init v9 (Autodesk Fusion 360 design; units mm, degrees)
Autodesk Fusion 360 part; units mm, degrees
sketch "Sketch1" plane through (0, 0, 0) normal (0, 0, 1) x (1, 0, 0)
  circle A0 centre (0, 0) radius 15
  circle A1 centre (0, 0) radius 20
  constraint coincident A0.centre A1.centre
extrude "Extrude1" add sketch "Sketch1" against normal blind 80 makes body 1
sketch "Sketch2" plane through (0, 0, 0) normal (0, 0, 1) x (1, 0, 0)
  circle A0 centre (0, 0) radius 15
  circle A1 centre (0, 0) radius 20
  circle A2 centre (0, 0) radius 50
  dimension "d5" = 100
  constraint concentric A0 A2
  measures "d5" diameter of A2
extrude "Extrude2" add sketch "Sketch2" along normal blind 10 separate body contours A2 makes body 2
extrude "Extrude3" add 1 faces at (39.7394, -3.4777, 10) along direction (0, 0, 1) blind 10 on bodies 2 bodies 2
chamfer "Chamfer1" distance 20 angle 45 1 edges at (-18.6465, 7.2323, 20) on bodies 2
sketch "Sketch3" plane through (0, 0, 20) normal (0, 0, 1) x (1, 0, 0)
  circle A0 centre (0, 0) radius 50
  circle A1 centre (0, 0) radius 40
  circle A2 centre (0, 0) radius 50
  constraint concentric A0 A2
extrude "Extrude4" add sketch "Sketch3" along normal blind 15 separate body contours A0 A2 | A1 makes body 3
sketch "Sketch4" plane through (0, 0, 20) normal (0, 0, -1) x (-1, 0, 0)
  circle A0 centre (0, 0) radius 50
  circle A1 centre (0, 0) radius 32.5
  dimension "d13" = 65
  constraint concentric A0 A1
  measures "d13" diameter of A1
extrude "Extrude5" add sketch "Sketch4" along normal blind 20 separate body contours A1 makes body 4
chamfer "Chamfer2" distance 20 angle 45 1 edges at (30.3006, -11.7525, 0) on bodies 4
sketch "Sketch5" plane through (0, 0, 35) normal (0, 0, 1) x (1, 0, 0)
  circle A0 centre (0, 0) radius 50
  circle A1 centre (35, 0) radius 1.5
  circle A2 centre (32.3358, 13.3939) radius 1.5
  circle A3 centre (24.7487, 24.7487) radius 1.5
  circle A4 centre (13.3939, 32.3358) radius 1.5
  circle A5 centre (0, 35) radius 1.5
  circle A6 centre (-13.3939, 32.3358) radius 1.5
  circle A7 centre (-24.7487, 24.7487) radius 1.5
  circle A8 centre (-32.3358, 13.3939) radius 1.5
  circle A9 centre (-35, 0) radius 1.5
  circle A10 centre (-32.3358, -13.3939) radius 1.5
  circle A11 centre (-24.7487, -24.7487) radius 1.5
  circle A12 centre (-13.3939, -32.3358) radius 1.5
  circle A13 centre (0, -35) radius 1.5
  circle A14 centre (13.3939, -32.3358) radius 1.5
  circle A15 centre (24.7487, -24.7487) radius 1.5
  circle A16 centre (32.3358, -13.3939) radius 1.5
  dimension "d18" = 3
  measures "d18" diameter of A1
extrude "Extrude6" cut sketch "Sketch5" against normal blind 70 contours A1 | A2 | A3 | A4 | A5 | A6 | A7 | A8 | A9 | A10 | A11 | A12 | A13 | A14 | A15 | A16 bodies 3
sketch "Sketch6" plane through (0, 0, 0) normal (0, 0, -1) x (-1, 0, 0)
  circle A0 centre (0, 0) radius 20
  circle A1 centre (0, 0) radius 50
  circle A2 centre (0, 0) radius 22.5
  dimension "d23" = 45
  constraint concentric A0 A2
  measures "d23" diameter of A2
extrude "Extrude7" add sketch "Sketch6" along normal blind 10 separate body contours A2 makes body 5
sketch "Sketch7" plane through (0, 0, 35) normal (0, 0, 1) x (1, 0, 0)
  circle A0 centre (0, -35) radius 1.5
  circle A1 centre (35, 0) radius 1.5
  circle A2 centre (0, 35) radius 1.5
  circle A3 centre (-35, 0) radius 1.5
  circle A4 centre (-32.3358, 13.3939) radius 1.5
  circle A5 centre (13.3939, 32.3358) radius 1.5
  circle A6 centre (32.3358, -13.3939) radius 1.5
  circle A7 centre (-13.3939, -32.3358) radius 1.5
  circle A8 centre (13.3939, -32.3358) radius 1.5
  circle A9 centre (32.3358, 13.3939) radius 1.5
  circle A10 centre (-13.3939, 32.3358) radius 1.5
  circle A11 centre (-32.3358, -13.3939) radius 1.5
  circle A12 centre (-24.7487, 24.7487) radius 1.5
  circle A13 centre (24.7487, 24.7487) radius 1.5
  circle A14 centre (24.7487, -24.7487) radius 1.5
  circle A15 centre (-24.7487, -24.7487) radius 1.5
  circle A16 centre (0, 0) radius 50
  circle A17 centre (0, 43.25) radius 4
sketch "Sketch8" plane through (0, 0, 20) normal (0, 0, -1) x (-1, 0, 0)
  circle A0 centre (0, -35) radius 1.5
  circle A1 centre (-35, 0) radius 1.5
  circle A2 centre (0, 35) radius 1.5
  circle A3 centre (35, 0) radius 1.5
  circle A4 centre (32.3358, 13.3939) radius 1.5
  circle A5 centre (-13.3939, 32.3358) radius 1.5
  circle A6 centre (-32.3358, -13.3939) radius 1.5
  circle A7 centre (13.3939, -32.3358) radius 1.5
  circle A8 centre (-13.3939, -32.3358) radius 1.5
  circle A9 centre (-32.3358, 13.3939) radius 1.5
  circle A10 centre (13.3939, 32.3358) radius 1.5
  circle A11 centre (32.3358, -13.3939) radius 1.5
  circle A12 centre (24.7487, 24.7487) radius 1.5
  circle A13 centre (-24.7487, 24.7487) radius 1.5
  circle A14 centre (-24.7487, -24.7487) radius 1.5
  circle A15 centre (24.7487, -24.7487) radius 1.5
  circle A16 centre (0, 0) radius 50
  circle A17 centre (0, 0) radius 40
  circle A18 centre (0, 0) radius 32.5
  dimension "d30" = 80
  dimension "d31" = 65
  constraint concentric A16 A17
  constraint concentric A16 A18
  measures "d30" diameter of A17
  measures "d31" diameter of A18
sketch "Sketch9" plane through (0, 0, 0) normal (1, 0, 0) x (0, 0, -1)
  line L0 (-20, 40) -> (-20, 36.5)
  line L1 (-20, 36.5) -> (-20, 40)
  line L2 (-20, 36.6244) -> (-20, 40)
  line L3 (-16.6454, 36.6244) -> (-20, 36.6244)
  line L4 (-16.6454, 36.6244) -> (-20, 40)
  constraint vertical L0
  constraint parallel L0 L1
  constraint coincident L0 L2.start
  constraint perpendicular L0 L3
revolve "Revolve1" add sketch "Sketch9" angle 360 about axis through (0, 0, 1.75) along (0, 0, 1) separate body makes body 6
sketch "Sketch10" plane through (0, 0, 0) normal (0, 0, -1) x (-1, 0, 0)
  circle A0 centre (0, 0) radius 12.5
  circle A1 centre (44, 0) radius 4
  circle A2 centre (31.1127, 31.1127) radius 4
  circle A3 centre (0, 44) radius 4
  circle A4 centre (-31.1127, 31.1127) radius 4
  circle A5 centre (-44, 0) radius 4
  circle A6 centre (-31.1127, -31.1127) radius 4
  circle A7 centre (0, -44) radius 4
  circle A8 centre (31.1127, -31.1127) radius 4
  dimension "d33" = 8
  measures "d33" diameter of A1
sketch "Sketch11" plane through (0, 0, 0) normal (0, 0, -1) x (-1, 0, 0)
  circle A0 centre (0, 0) radius 20
  circle A1 centre (0, 0) radius 50
  circle A2 centre (0, 0) radius 79
  dimension "d36" = 158
  constraint concentric A0 A2
  measures "d36" diameter of A2
extrude "Extrude8" add sketch "Sketch11" against normal blind 20 contours A2 bodies 2
sketch "Sketch12" plane through (0, 0, 35) normal (0, 0, 1) x (1, 0, 0)
  circle A0 centre (0, -35) radius 1.5
  circle A1 centre (35, 0) radius 1.5
  circle A2 centre (0, 35) radius 1.5
  circle A3 centre (-35, 0) radius 1.5
  circle A4 centre (-32.3358, 13.3939) radius 1.5
  circle A5 centre (13.3939, 32.3358) radius 1.5
  circle A6 centre (32.3358, -13.3939) radius 1.5
  circle A7 centre (-13.3939, -32.3358) radius 1.5
  circle A8 centre (13.3939, -32.3358) radius 1.5
  circle A9 centre (32.3358, 13.3939) radius 1.5
  circle A10 centre (-13.3939, 32.3358) radius 1.5
  circle A11 centre (-32.3358, -13.3939) radius 1.5
  circle A12 centre (-24.7487, 24.7487) radius 1.5
  circle A13 centre (24.7487, 24.7487) radius 1.5
  circle A14 centre (24.7487, -24.7487) radius 1.5
  circle A15 centre (-24.7487, -24.7487) radius 1.5
  circle A16 centre (0, 0) radius 50
  circle A17 centre (0, 0) radius 79
  circle A18 centre (0, 0) radius 50
  dimension "d39" = 158
  constraint concentric A16 A17
  constraint concentric A16 A18
  measures "d39" diameter of A17
extrude "Extrude9" add sketch "Sketch12" against normal blind 15 separate body contours A17 makes body 7
sketch "Sketch13" plane through (0, 0, 35) normal (0, 0, 1) x (1, 0, 0)
  circle A0 centre (0, 0) radius 50
  circle A1 centre (0, 0) radius 79
  line L0 (0, 0) -> (79, 0) construction
  line L1 (0, 0) -> (79, 0) construction
  circle A2 centre (-59.7558, -34.5) radius 8.5
  circle A3 centre (59.7558, -34.5) radius 8.5
  circle A4 centre (0, 69) radius 8.5
  point P0 (-79, 0)
  dimension "d52" = 360
  constraint horizontal L0
  constraint coincident A0.centre A1.centre
  constraint horizontal L1
extrude "Extrude10" cut sketch "Sketch13" against normal blind 90 contours A2 | A3 | A4 bodies 2 7
sketch "Sketch14" plane through (0, 0, 0) normal (1, 0, 0) x (0, 0, -1)
  line L0 (-35, 0) -> (-20, 0)
  line L1 (-20, 0) -> (-20, 50)
  line L2 (-20, 50) -> (-23.3513, 50)
  line L3 (-23.3513, 50) -> (-23.3513, 40)
  line L4 (-23.3513, 40) -> (-20, 40)
  line L5 (-20, 50) -> (-23.3513, 50)
  constraint horizontal L0
  constraint perpendicular L0 L1
  constraint perpendicular L1 L2
  constraint perpendicular L2 L3
  constraint coincident L1 L4.end
  constraint perpendicular L1 L4
revolve "Revolve2" add sketch "Sketch14" angle 360 about axis through (0, 0, 1.75) along (0, 0, 1) separate body makes body 8
revolve "Revolve3" cut sketch "Sketch14" angle 360 about axis through (0, 0, 1.75) along (0, 0, 1) bodies 3
equation "d31 = ( 32.5 * 2 ) * 1 mm"
equation "d39 = ( 79 * 2 ) * 1 mm"
named bodies: "Barrel", "MountFlange", "FaceDie", "BarrelNut", "MountFlange-Revolve"
